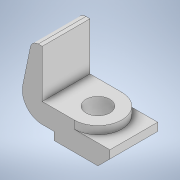
# Autodesk Inventor part: ch4-3
Saved by Autodesk Inventor 2020 (Build 240168000, 168)
## iProperties
Created: 2020-02-07
Part Number: ch4-3
Material: Generic
Document SubType Name: Modeling
Designer: Eric
Mass: 457.286 g
Surface Area: 525.614 cm^2
Volume: 457.286 cm^3
Density: 1 g/cm^3
Appearance: Default
Author: Eric
Autodesk Inventor part; units mm, degrees
ref_plane "YZ Plane" through (0, 0, 0) normal (1, 0, 0) x (0, 1, 0)
ref_plane "XZ Plane" through (0, 0, 0) normal (0, 1, 0) x (-1, 0, 0)
ref_plane "XY Plane" through (0, 0, 0) normal (0, 0, 1) x (1, 0, 0)
sketch "Sketch1" plane through (0, 0, 0) normal (0, 0, 1) x (1, 0, 0)
  line L0 (0, 76.2) -> (0, 0)
  line L1 (0, 0) -> (50.8, 0)
  line L2 (50.8, 0) -> (50.8, -12.7)
  line L3 (50.8, -12.7) -> (107.95, -12.7)
  line L4 (107.95, -12.7) -> (107.95, -25.4)
  line L5 (107.95, -25.4) -> (88.9, -44.45)
  line L6 (88.9, -44.45) -> (19.05, -44.45)
  line L7 (0, 76.2) -> (-6.35, 76.2)
  circle A0 centre (-6.35, 63.5) radius 12.7
  circle A1 centre (0, 0) radius 31.75
  line L8 (19.05, -44.45) -> (19.05, -31.75)
  line L9 (-31.0951, 6.4155) -> (-18.788, 66.0662)
  line L10 (19.05, -31.75) -> (0, -31.75)
  point P0 (0, 74.4985)
  dimension "d0" = 6.35
  dimension "d1" = 69.85
  dimension "d2" = 12.7
  dimension "d3" = 76.2
  dimension "d4" = 63.5
  dimension "d5" = 19.05
  dimension "d7" = 31.75
  dimension "d8" = 107.95
  dimension "d9" = 25.4
  dimension "d10" = 12.7
  dimension "d11" = 50.8
  dimension "d12" = 44.45
  constraints: 22 end point, 4 perpendicular, 4 point on circle, 3 tangent, 2 centre point, 2 coincident, 2 horizontal, 2 vertical, 1 parallel
  measures "d0" distance of L0.start L7.end
  measures "d1" distance of L5.end L6.end
  measures "d2" distance of L3.end L4.end
  measures "d3" distance of L0.start L0.end
  measures "d4" diameter of A1
  measures "d5" distance of L8.end L10.end
  measures "d7" distance between parallel lines of L1 L10
  measures "d8" horizontal distance of L3.end L0.start
  measures "d9" diameter of A0
  measures "d10" distance of L1.end L2.end
  measures "d11" distance of L1.end point (0, 0)
  measures "d12" distance between parallel lines of L1 L6
extrude "Extrusion1" add sketch "Sketch1" along normal blind 76.2 contours L0 A0 L7 | L0 A0 | L0 A1 L9 A0 | L0 L1 A1 | L1 L2 L3 L4 L5 L6 L8 L10 A1 picked at (-6.7952, 59.4597) picked at (-19.9789, 6.5634)
sketch "Sketch2" plane through (50.8, -12.7, 0) normal (0, 1, 0) x (1, 0, 0)
  line L0 (0, 0) -> (0, -76.2) construction
  circle A0 centre (0, -38.1) radius 38.1
  point P0 (-50.8, 0)
  constraints: 1 midpoint, 1 vertical alignment, 2 other
extrude "Extrusion2" add sketch "Sketch2" along normal up to surface (12.7 mm away)
sketch "Sketch3" plane through (0, 0, 76.2) normal (0, 1, 0) x (1, 0, 0)
  arc A0 (50.8, 0) -> (50.8, 76.2) centre (50.8, 38.1) ccw construction
  point P0 (0, 76.2)
  constraints: 1 coincident
hole "Hole1" at (50.8, 0, 38.1) direction (0, -1, 0) diameter 38.1 end through all
body "Solid1"
